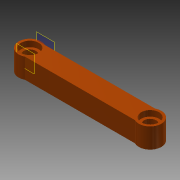
# Autodesk Inventor part: xy wall arm SP
Saved by Autodesk Inventor 2014 (Build 180170000, 170)
## iProperties
Created: 2013-07-22
Part Number: xy wall arm SP
Material: Generic
Document SubType Name: Modeling
Designer: employee
Density: 1 g/cm^3
Mass: 93.7054 g
Surface Area: 211.467 cm^2
Volume: 93.7054 cm^3
Appearance: Smooth - Light Orange
Author: employee
Autodesk Inventor part; units mm, degrees
ref_plane "YZ Plane" through (0, 0, 0) normal (1, 0, 0) x (0, 1, 0)
ref_plane "XZ Plane" through (0, 0, 0) normal (0, 1, 0) x (-1, 0, 0)
ref_plane "XY Plane" through (0, 0, 0) normal (0, 0, 1) x (1, 0, 0)
sketch "Sketch1" plane through (0, 0, 0) normal (0, 0, 1) x (1, 0, 0)
  line L0 (0, 12.5) -> (149.8, 12.5)
  arc A0 (149.8, -12.5) -> (149.8, 12.5) centre (149.8, 0) ccw
  line L1 (149.8, -12.5) -> (0, -12.5)
  arc A1 (0, 12.5) -> (0, -12.5) centre (0, 0) ccw
  dimension "d0" = 149.8
  dimension "d2" = 12.5
  constraints: 4 end point, 4 point on circle, 4 tangent, 2 centre point, 1 coincident, 1 horizontal, 1 parallel
  measures "d0" distance of L0.start L0.end
  measures "d2" radius of A1
extrude "Extrusion1" add sketch "Sketch1" along normal blind 25
sketch "Sketch2" plane through (0, 0, 25) normal (0, 0, 1) x (1, 0, 0)
  arc A0 (0, 12.5) -> (0, -12.5) centre (0, 0) ccw projected
  arc A1 (149.8, -12.5) -> (149.8, 12.5) centre (149.8, 0) ccw projected
  circle A2 centre (0, 0) radius 7.55
  circle A3 centre (149.8, 0) radius 7.55
  dimension "d5" = 15.1
  constraints: 2 centre point, 2 coincident, 1 equal radius
  measures "d5" diameter of A3
extrude "Extrusion2" cut sketch "Sketch2" against normal through all
sketch "Sketch3" plane through (0, 0, 25) normal (0, 0, 1) x (1, 0, 0)
  circle A0 centre (0, 0) radius 7.55 projected
  circle A1 centre (149.8, 0) radius 7.55 projected
  arc A2 (0, 12.5) -> (0, -12.5) centre (0, 0) ccw projected
  arc A3 (149.8, -12.5) -> (149.8, 12.5) centre (149.8, 0) ccw projected
  circle A4 centre (0, 0) radius 11.05
  circle A5 centre (149.8, 0) radius 11.05
  dimension "d9" = 22.1
  constraints: 2 centre point, 2 coincident, 1 equal radius
  measures "d9" diameter of A5
extrude "Extrusion3" cut sketch "Sketch3" against normal blind 7
sketch "Sketch4" plane through (0, 0, 0) normal (0, 0, -1) x (-1, 0, 0)
  circle A0 centre (0, 0) radius 7.55 projected
  circle A1 centre (-149.8, 0) radius 7.55 projected
  circle A2 centre (-149.8, 0) radius 11.05 projected
  circle A3 centre (0, 0) radius 11.05 projected
extrude "Extrusion4" cut sketch "Sketch4" against normal blind 7
chamfer "Chamfer1" distance 3.5 angle 45 2 edges at (142.25, 0, 7) (-7.55, 0, 7)
sketch "Sketch5" plane through (0, 0, 25) normal (0, 0, 1) x (1, 0, 0)
  circle A0 centre (0, 0) radius 11.05 projected
  circle A1 centre (149.8, 0) radius 11.05 projected
  arc A2 (0, 12.5) -> (0, -12.5) centre (0, 0) ccw projected
  arc A3 (149.8, -12.5) -> (149.8, 12.5) centre (149.8, 0) ccw projected
  circle A4 centre (0, 0) radius 14.05
  circle A5 centre (149.8, 0) radius 14.05
  dimension "d18" = 3
  constraints: 2 centre point, 2 coincident, 1 equal radius
  measures "d18" radial gap between concentric circles of A1 A5
extrude "Extrusion5" add sketch "Sketch5" against normal up to surface (25 mm away)
ref_plane "Work Plane2" through (6.8813, -12.5, 23) normal (0, -1, 0) x (1, 0, 0)
sketch "Sketch6" plane through (6.415, -12.5, 0) normal (0, -1, 0) x (1, 0, 0)
  line L0 (0, 0) -> (136.97, 2.0217)
  line L1 (136.97, 2.0217) -> (131.3954, 22.9783)
  line L2 (0, 25) -> (136.97, 25) construction
  line L3 (136.97, 25) -> (136.97, 0) construction
  line L4 (136.97, 0) -> (0, 0) construction
  line L5 (0, 0) -> (0, 25) construction
  line L6 (136.97, 0) -> (136.97, 25) projected
  line L7 (0, 25) -> (136.97, 25) projected
  point P0 (-6.8813, -23)
  point P1 (136.97, 12.5)
  point P2 (134.1827, 12.5)
  point P3 (68.485, 25)
  point P4 (68.485, 1.0109)
  constraints: 6 midpoint, 4 end point, 1 horizontal alignment, 1 vertical alignment, 2 other
ref_plane "Work Plane1" through (6.8813, 12.5, 23) normal (0, 1, 0) x (1, 0, 0)
sketch "Sketch7" plane through (6.8813, 12.5, 23) normal (0, 1, 0) x (1, 0, 0)
  line L0 (136.5037, 23) -> (-0.4663, 23) construction
  line L1 (-0.4663, 23) -> (-0.4663, -2) construction
  line L2 (-0.4663, -2) -> (136.5037, -2) construction
  line L3 (136.5037, -2) -> (136.5037, 23) construction
  line L4 (136.5037, -2) -> (136.5037, 23) projected
  line L5 (-0.4663, 23) -> (136.5037, 23) projected
  line L6 (-0.4663, 23) -> (-0.4663, -2) projected
  line L7 (136.5037, -2) -> (-0.4663, -2) projected
  point P0 (-6.8813, 23)
  constraints: 2 coincident, 2 other
extrude "Extrusion6" [suppressed]
extrude "Extrusion7" [suppressed]
body "Solid1"
